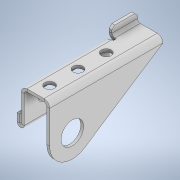
# Autodesk Inventor part: 26886-Vodička_Vojtěch_příklad-5
Saved by Autodesk Inventor 2022 (Build 260153000, 153)
## iProperties
Created: 2022-03-24
Part Number: 26886-Vodička_Vojtěch_příklad-5
Material: Všeobecné
Document SubType Name: Sheet Metal
Designer: vojta
Density: 1 g/cm^3
Sheet Metal Rule: Výchozí_mm
Appearance: Výchozí
Author: vojta
Autodesk Inventor part; units mm, degrees
ref_plane "YZ Plane" through (0, 0, 0) normal (1, 0, 0) x (0, 1, 0)
ref_plane "XZ Plane" through (0, 0, 0) normal (0, 1, 0) x (-1, 0, 0)
ref_plane "XY Plane" through (0, 0, 0) normal (0, 0, 1) x (1, 0, 0)
sketch "Náčrt1" plane through (0, 0, 0) normal (0, 1, 0) x (-1, 0, 0)
  line L0 (0, 0) -> (0, -80)
  line L1 (0, -80) -> (20, -80)
  line L2 (0, 0) -> (20, 0)
  line L3 (20, 0) -> (20, -60)
  line L4 (20, -60) -> (15, -60)
  line L5 (15, -60) -> (15, -62)
  line L6 (15, -62) -> (20, -62)
  line L7 (20, -62) -> (20, -80)
  circle A0 centre (10, -10) radius 3.5
  circle A1 centre (10, -30) radius 3.5
  circle A2 centre (10, -50) radius 3.5
  dimension "d0" = 80
  dimension "d1" = 20
  dimension "d2" = 20
  dimension "d3" = 60
  dimension "d4" = 5
  dimension "d5" = 2
  dimension "d6" = 5
  dimension "d34" = 7
  dimension "d35" = 7
  dimension "d36" = 7
  measures "d0" distance of L0.start L0.end
  measures "d1" distance of L0.end L1.end
  measures "d2" distance of L0.start L2.end
  measures "d3" distance of L2.end L3.end
  measures "d4" distance of L3.end L4.end
  measures "d5" distance of L4.end L5.end
  measures "d6" distance of L5.end L6.end
  measures "d34" diameter of A0
  measures "d35" diameter of A1
  measures "d36" diameter of A2
extrude "Deska4" add sketch "Náčrt1" along normal blind 2
sketch "Náčrt4" plane through (-18, 0, -62) normal (-1, 0, 0) x (0, -1, 0)
  line L0 (0, -18) -> (0, 0)
  line L1 (0, 0) -> (-8, 0)
  line L2 (-8, 0) -> (-8, -18)
  line L3 (-8, -18) -> (0, -18)
  constraints: 6 end point, 1 horizontal, 1 perpendicular, 1 vertical
edge flange "Obruba3" height 6 angle 90 thickness 2 bend radius 2 thickness toward (-1, 0, 0) relief straight relief width 2 relief depth 1 edges at (-20, 2, -71) wall of the first edge with corners at (-18, 0, -80) (-18, 0, -62) (-18, 8, -62) (-18, 8, -80)
bend "Ohyb3"
corner "Roh3"
chamfer "Zkosení rohu2" distance 2 angle 45 2 edges at (-19, 8, -80) (-19, 8, -62)
sketch "Náčrt5" plane through (-18, 2, -60) normal (-1, 0, 0) x (0, -1, 0)
  line L0 (0, 60) -> (0, 0)
  line L1 (0, 0) -> (26, 0)
  line L2 (26, 0) -> (26, 60)
  line L3 (26, 60) -> (0, 60)
  constraints: 6 end point, 1 horizontal, 1 perpendicular, 1 vertical
edge flange "Obruba4" height 26 angle 90 thickness 2 bend radius 2 thickness toward (-1, 0, 0) relief straight relief width 2 relief depth 1 edges at (-20, 0, -30) wall of the first edge with corners at (-18, 2, 0) (-18, 2, -60) (-18, -24, -60) (-18, -24, 0)
bend "Ohyb4"
corner "Roh4"
sketch "Náčrt6" plane through (-20, -21.5, -60) normal (0, 0, -1) x (-1, 0, 0)
  line L0 (-2, 0) -> (0, 0)
  arc A0 (0, 0) -> (1, 0) centre (0.5, 0) ccw
  line L1 (1, 0) -> (1, 5.5)
  line L2 (1, 5.5) -> (3, 5.5)
  line L3 (3, 5.5) -> (3, 0)
  arc A1 (-2, 0) -> (3, 0) centre (0.5, 0) ccw
  constraints: 8 end point, 4 point on circle
hem "Lem1" sketch "Náčrt6" thickness 2 along (0, 0, 1) edges at (-20, -24, -30)
sketch "Náčrt7" plane through (-18, -2, 0) normal (1, 0, 0) x (0, 0, -1)
  line L0 (13, -11) -> (47, -11)
  line L1 (60, -19.5) -> (60, 0) projected
  line L2 (13, -3) -> (47, -3)
  line L3 (10, -6) -> (10, -8)
  line L4 (50, -6) -> (50, -8)
  line L5 (0, 0) -> (0, -19.5) projected
  arc A0 (13, -3) -> (10, -6) centre (13, -6) ccw
  arc A1 (10, -8) -> (13, -11) centre (13, -8) ccw
  arc A2 (47, -11) -> (50, -8) centre (47, -8) ccw
  arc A3 (50, -6) -> (47, -3) centre (47, -6) ccw
  point P0 (0, 2)
  dimension "d72" = 40
  dimension "d73" = 10
  dimension "d74" = 8
  dimension "d75" = 5
  dimension "d76" = 3
  constraints: 8 end point, 8 point on circle, 8 tangent, 4 centre point, 3 equal radius, 2 perpendicular, 1 horizontal
  measures "d72" distance between parallel lines of L4 L3
  measures "d73" distance between parallel lines of L5 L3
  measures "d74" distance between parallel lines of L0 L2
  measures "d75" distance from line of point (0, 2) L2
  measures "d76" radius of A0
extrude "Vyříznutí1" cut sketch "Náčrt7" against normal blind 2
sketch "Náčrt8" plane through (-2, 2, 0) normal (1, 0, 0) x (0, 1, 0)
  line L0 (0, -80) -> (0, 0)
  line L1 (0, 0) -> (-43, 0)
  line L2 (-43, 0) -> (-43, -80)
  line L3 (-43, -80) -> (0, -80)
  constraints: 6 end point, 1 horizontal, 1 perpendicular, 1 vertical
edge flange "Obruba5" height 43 angle 90 thickness 2 bend radius 2 thickness toward (1, 0, 0) relief straight relief width 2 relief depth 1 edges at (0, 0, -40) wall of the first edge with corners at (-2, 2, -80) (-2, 2, 0) (-2, -41, 0) (-2, -41, -80)
bend "Ohyb5"
corner "Roh5"
sketch "Náčrt9" plane through (0, -41, 0) normal (1, 0, 0) x (0, 0, -1)
  line L0 (60, 17) -> (0, 17) projected
  line L1 (80, 0) -> (0, 0) projected
  circle A0 centre (16, 16) radius 8
  point P0 (0, 41)
  point P1 (80, 41)
  dimension "d90" = 16
  constraints: 1 centre point
  measures "d90" diameter of A0
extrude "Vyříznutí2" cut sketch "Náčrt9" against normal blind 2
sketch "Náčrt10" plane through (0, -41, 0) normal (1, 0, 0) x (0, 0, -1)
  circle A0 centre (16, 16) radius 8 projected
  arc A1 (0, 16) -> (25.132, 2.862) centre (16, 16) ccw
  line L0 (80, 41) -> (0, 41) projected
  line L1 (0, 17) -> (0, 19.5) projected
  line L2 (0, 39) -> (0, 0) projected
  line L3 (0, 16) -> (0, 0)
  line L4 (80, 0) -> (0, 0) projected
  line L5 (0, 0) -> (80, 0)
  line L6 (62, 41) -> (80, 41) projected
  line L7 (80, 0) -> (80, 39)
  line L8 (0, 39) -> (80, 39) projected
  line L9 (25.132, 2.862) -> (80, 39)
  point P0 (16, 0)
  point P1 (16, 0)
  dimension "d93" = 32
  constraints: 8 end point, 4 point on circle, 2 point on line, 1 centre point, 1 coincident, 1 horizontal, 1 perpendicular, 1 vertical
  measures "d93" diameter of A1
extrude "Vyříznutí4" cut sketch "Náčrt10" against normal blind 2 contours A1 L4 L2 | A1 L9 L7 L4
equation "\"d37\" = Tloušťka"
equation "\"d61\" = ŠířkaVýštipu"
equation "\"d62\" = HloubkaVýštipu"
equation "\"d63\" = MinimálníZbytek"
equation "\"d64\" = PřechodovýPoloměr"
equation "\"d65\" = 4 * Tloušťka"
equation "\"d66\" = 0.5 * Tloušťka"
equation "\"d67\" = 0.5 * d66"
equation "\"d77\" = Tloušťka"
equation "\"d91\" = Tloušťka"
equation "\"d96\" = Tloušťka"
equation "\"d38\" = ŠířkaVýštipu"
equation "\"d39\" = HloubkaVýštipu"
equation "\"d40\" = MinimálníZbytek"
equation "\"d41\" = PřechodovýPoloměr"
equation "\"d44\" = PoloměrOhybu"
equation "\"d45\" = VelikostRohovéhoVýštipu"
equation "\"d46\" = VelikostMezery"
equation "\"d47\" = VelikostJacobihoPoloměru"
equation "\"d51\" = ŠířkaVýštipu"
equation "\"d52\" = HloubkaVýštipu"
equation "\"d53\" = MinimálníZbytek"
equation "\"d54\" = PřechodovýPoloměr"
equation "\"d57\" = PoloměrOhybu"
equation "\"d58\" = VelikostRohovéhoVýštipu"
equation "\"d59\" = VelikostMezery"
equation "\"d60\" = VelikostJacobihoPoloměru"
equation "\"d79\" = ŠířkaVýštipu"
equation "\"d80\" = HloubkaVýštipu"
equation "\"d81\" = MinimálníZbytek"
equation "\"d82\" = PřechodovýPoloměr"
equation "\"d85\" = PoloměrOhybu"
equation "\"d86\" = VelikostRohovéhoVýštipu"
equation "\"d87\" = VelikostMezery"
equation "\"d88\" = VelikostJacobihoPoloměru"
equation "\"PoloměrOhybu\" = Tloušťka"
equation "\"ŠířkaVýštipu\" = Tloušťka"
equation "\"HloubkaVýštipu\" = 0.5 * Tloušťka"
equation "\"VelikostRohovéhoVýštipu\" = 4 * Tloušťka"
equation "\"MinimálníZbytek\" = 2 * Tloušťka"
equation "\"PřechodovýPoloměr\" = PoloměrOhybu"
equation "\"VelikostJacobihoPoloměru\" = PoloměrOhybu"
equation "\"VelikostMezery\" = Tloušťka"
equation "\"Tloušťka\" = 2"
